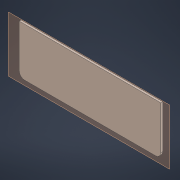
# Autodesk Inventor part: NEW_COVER_220DET_SMALL_COVER
Saved by Autodesk Inventor 2021 (Build 250183000, 183)
## iProperties
Created: 2020-07-15
Part Number: NEW_COVER_220DET_SMALL_COVER
Material: Generic
Document SubType Name: Modeling
Designer: erwin
Density: 1 g/cm^3
Appearance: Default
Author: erwin
Autodesk Inventor part; units mm, degrees
ref_plane "YZ Plane" through (0, 0, 0) normal (1, 0, 0) x (0, 1, 0)
ref_plane "XZ Plane" through (0, 0, 0) normal (0, 1, 0) x (-1, 0, 0)
ref_plane "XY Plane" through (0, 0, 0) normal (0, 0, 1) x (1, 0, 0)
ref_plane "Work Plane1" through (0, 0, 0) normal (0, 0, 1) x (1, 0, 0)
sketch "Sketch1" plane through (0, 0, 0) normal (0, 0, 1) x (1, 0, 0)
  line L0 (54.9687, 15.1484) -> (54.9687, -17.3516) projected
  arc A0 (50.9687, -21.3516) -> (54.9687, -17.3516) centre (50.9687, -17.3516) ccw projected
  line L1 (50.9687, -21.3516) -> (-24.2638, -21.3516) projected
  line L2 (54.9687, -22.8516) -> (-24.2638, -22.8516) projected
  arc A1 (54.9687, -22.8516) -> (55.9687, -21.8516) centre (54.9687, -21.8516) ccw projected
  line L3 (55.9687, 15.1484) -> (55.9687, -21.8516) projected
  line L4 (54.9687, 15.1484) -> (55.9687, 15.1484) projected
  line L5 (-51.5313, 15.1484) -> (54.9687, 15.1484)
  line L6 (-24.2638, -21.3516) -> (-24.2638, -22.8516) projected
  line L7 (-39.2638, -22.8516) -> (-39.2638, -21.3516) projected
  line L8 (-39.2638, -21.3516) -> (-47.5313, -21.3516) projected
  arc A2 (-51.5313, -17.3516) -> (-47.5313, -21.3516) centre (-47.5313, -17.3516) ccw projected
  line L9 (-51.5313, -17.3516) -> (-51.5313, 15.1484) projected
  line L10 (-54.0313, 15.1484) -> (-51.5313, 15.1484) projected
  line L11 (-54.0313, -21.8516) -> (-54.0313, 15.1484) projected
  arc A3 (-54.0313, -21.8516) -> (-53.0313, -22.8516) centre (-53.0313, -21.8516) ccw projected
  line L12 (-39.2638, -22.8516) -> (-53.0313, -22.8516) projected
  line L13 (-39.2638, -21.3516) -> (-24.2638, -21.3516)
  point P0 (0, 0)
  constraints: 4 end point, 2 horizontal
extrude "Extrusion1" add sketch "Sketch1" against normal blind 1.5 contours L0 A0 L1 L13 L8 A2 L9 L5
thicken "Thicken1" operation add thickness 0.1 both sides no extend neighbours yes toward (-1, 0, 0) faces at (54.9687, -6.5183, -0.5) (53.222, -20.6566, -1) (0.8137, -21.3516, -0.5) (-34.2638, -21.3516, -0.5) (-44.7755, -21.3516, -0.5) (-50.4635, -20.0723, -1) (-51.5313, 4.3151, -0.5)
body "Solid1"
